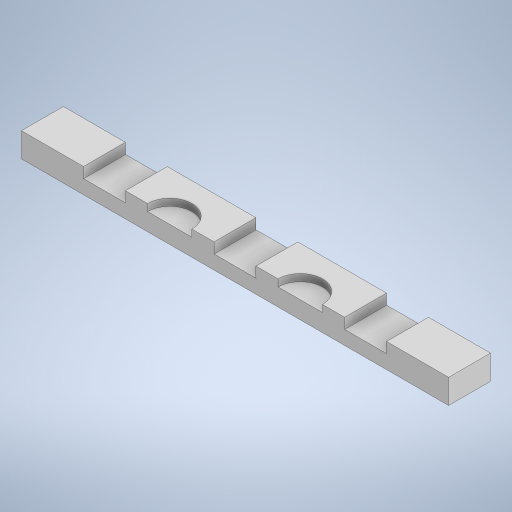
# Autodesk Inventor part: Button Support
Saved by Autodesk Inventor 2023.1 (Build 271208000, 208)
## iProperties
Created: 2022-10-10
Part Number: Button Support
Material: Generic
Document SubType Name: Modeling
Designer: nicol
Density: 1 g/cm^3
Appearance: Default
Author: nicol
Autodesk Inventor part; units mm, degrees
ref_plane "YZ Plane" through (0, 0, 0) normal (1, 0, 0) x (0, 1, 0)
ref_plane "XZ Plane" through (0, 0, 0) normal (0, 1, 0) x (-1, 0, 0)
ref_plane "XY Plane" through (0, 0, 0) normal (0, 0, 1) x (1, 0, 0)
sketch "Sketch1" plane through (0, 0, 0) normal (0, 0, 1) x (1, 0, 0)
  line L0 (0, 0) -> (61.18, 0)
  line L1 (61.18, 0) -> (61.18, 2)
  line L2 (61.18, 2) -> (0, 2)
  line L3 (0, 2) -> (0, 0)
  line L4 (14.89, 2) -> (27.59, 2)
  line L5 (27.59, 2) -> (27.59, 3.5)
  line L6 (27.59, 3.5) -> (14.89, 3.5)
  line L7 (14.89, 3.5) -> (14.89, 2)
  line L8 (33.59, 2) -> (46.29, 2)
  line L9 (46.29, 2) -> (46.29, 3.5)
  line L10 (46.29, 3.5) -> (33.59, 3.5)
  line L11 (33.59, 3.5) -> (33.59, 2)
  line L12 (8.89, 2) -> (0, 2)
  line L13 (0, 2) -> (0, 3.5)
  line L14 (0, 3.5) -> (8.89, 3.5)
  line L15 (8.89, 3.5) -> (8.89, 2)
  line L16 (52.29, 2) -> (61.18, 2)
  line L17 (61.18, 2) -> (61.18, 3.5)
  line L18 (61.18, 3.5) -> (52.29, 3.5)
  line L19 (52.29, 3.5) -> (52.29, 2)
  dimension "d0" = 6
  dimension "d1" = 2
  dimension "d2" = 1.5
  dimension "d3" = 6
  dimension "d4" = 6
  dimension "d5" = 12.7
  dimension "d6" = 8.89
  dimension "d7" = 8.89
  constraints: 40 end point, 10 parallel, 9 collinear, 5 horizontal, 5 perpendicular, 1 point on line
  measures "d0" distance between parallel lines of L5 L11
  measures "d1" distance of L0.end L1.end
  measures "d2" distance of L4.end L5.end
  measures "d3" distance between parallel lines of L19 L9
  measures "d4" distance between parallel lines of L15 L7
  measures "d5" distance of L5.end L6.end
  measures "d6" distance of L17.end L18.end
  measures "d7" distance of L13.end L14.end
extrude "Extrusion1" add sketch "Sketch1" along normal blind 6
sketch "Sketch2" plane through (14.89, 3.5, 0) normal (0, 1, 0) x (1, 0, 0)
  line L0 (31.4, 0) -> (18.7, 0) projected
  line L1 (18.7, 0) -> (18.7, -6) projected
  line L2 (31.4, -6) -> (18.7, -6) projected
  line L3 (31.4, 0) -> (31.4, -6) projected
  line L4 (12.7, 0) -> (0, 0) projected
  line L5 (0, 0) -> (0, -6) projected
  line L6 (12.7, -6) -> (0, -6) projected
  line L7 (12.7, 0) -> (12.7, -6) projected
  line L8 (-14.89, -6) -> (46.29, -6) projected
  circle A0 centre (6.35, -6) radius 3.175
  circle A1 centre (25.05, -6) radius 3.175
  point P0 (-14.89, 0)
  point P1 (21.875, -6)
  point P2 (28.225, -6)
  point P3 (3.175, -6)
  point P4 (9.525, -6)
  dimension "d10" = 6.35
  dimension "d11" = 6.35
  constraints: 2 centre point, 2 midpoint, 1 point on line
  measures "d10" diameter of A0
  measures "d11" diameter of A1
extrude "Extrusion2" cut sketch "Sketch2" against normal blind 1 contours L2 A1 | L6 A0 picked at (25.8422, -4.7916) picked at (7.1422, -4.7916)
body "Solid1"
